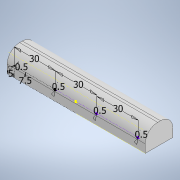
# Autodesk Inventor part: actuator_tube
Saved by Autodesk Inventor 2021 (Build 250183000, 183)
## iProperties
Created: 2021-04-28
Part Number: actuator_tube
Material: Generic
Document SubType Name: Modeling
Designer: Charlie
Density: 1 g/cm^3
Appearance: Default
Author: Charlie
Autodesk Inventor part; units mm, degrees
ref_plane "YZ Plane" through (0, 0, 0) normal (1, 0, 0) x (0, 1, 0)
ref_plane "XZ Plane" through (0, 0, 0) normal (0, 1, 0) x (-1, 0, 0)
ref_plane "XY Plane" through (0, 0, 0) normal (0, 0, 1) x (1, 0, 0)
sketch "Sketch1" plane through (0, 0, 0) normal (0, 0, 1) x (1, 0, 0)
  line L0 (-50, 7.5) -> (50, 7.5)
  line L1 (50, 7.5) -> (50, -7.5)
  line L2 (50, -7.5) -> (-50, -7.5)
  line L3 (-50, -7.5) -> (-50, 7.5)
  line L4 (-50, 7.5) -> (50, -7.5) construction
  line L5 (50, 7.5) -> (-50, -7.5) construction
  point P0 (0, 0)
  dimension "d0" = 100
  dimension "d1" = 15
  constraints: 12 end point, 2 midpoint, 2 parallel, 1 horizontal, 1 perpendicular
  measures "d0" distance of L1.end L2.end
  measures "d1" distance of L0.end L1.end
extrude "Extrusion1" add sketch "Sketch1" along normal blind 20
sketch "Sketch2" plane through (-50, -7.5, 0) normal (-1, 0, 0) x (0, 0, 1)
  line L0 (0, 0) -> (0, 15) projected
  line L1 (0, 0) -> (20, 0)
  line L2 (20, 0) -> (20, 15) projected
  line L3 (20, 0) -> (20, 6)
  line L4 (11, 15) -> (9, 15)
  line L5 (0, 6) -> (0, 0)
  arc A0 (9, 15) -> (0, 6) centre (9, 6) ccw
  arc A1 (20, 6) -> (11, 15) centre (11, 6) ccw
  point P0 (0, 7.5)
  dimension "d4" = 9
  dimension "d10" = 20
  dimension "d11" = 15
  constraints: 8 end point, 4 point on circle, 4 tangent, 3 perpendicular, 2 centre point, 2 point on line, 1 equal radius
  measures "d4" radius of A0
  measures "d10" distance of L0.start L1.end
  measures "d11" distance of L1.end L2.end
extrude "Extrusion2" cut sketch "Sketch2" against normal through all keep common part
shell "Shell1" thickness 1 removed faces 1 at (-50, 1.5, 10.3333)
extrude "Extrusion3" add sketch "Sketch2" against normal blind 1
sketch "Sketch3" plane through (0, 0, 20) normal (0, 0, 1) x (1, 0, 0)
  line L0 (-50, -7.5) -> (50, -7.5) construction
  line L1 (-50, -7.5) -> (0, -7.5) construction
  line L2 (-50, -7.5) -> (-45, -7.5) construction
  line L3 (-45, -7.5) -> (-45, 7.5) construction
  line L4 (-49, 6.5) -> (49, 6.5) construction
  circle A0 centre (-45, 0) radius 0.25
  line L5 (-45, 0) -> (-15, 0) construction
  circle A1 centre (-15, 0) radius 0.25
  line L6 (-15, 0) -> (15, 0) construction
  circle A2 centre (15, 0) radius 0.25
  line L7 (15, 0) -> (45, 0) construction
  circle A3 centre (45, 0) radius 0.25
  point P0 (0, 0)
  dimension "d12" = 5
  dimension "d13" = 0.5
  dimension "d14" = 30
  dimension "d15" = 0.5
  dimension "d16" = 7.5
  dimension "d17" = 30
  dimension "d18" = 0.5
  dimension "d19" = 30
  dimension "d20" = 0.5
  constraints: 12 end point, 4 centre point, 3 coincident, 3 horizontal, 2 midpoint, 1 perpendicular, 1 point on line
  measures "d12" distance of L0.start L2.end
  measures "d13" diameter of A0
  measures "d14" distance of L5.start L5.end
  measures "d15" diameter of A1
  measures "d16" distance between parallel lines of L0 L5
  measures "d17" distance of L6.start L6.end
  measures "d18" diameter of A2
  measures "d19" distance of L7.start L7.end
  measures "d20" diameter of A3
body "Solid1"
